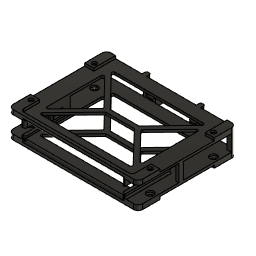
BatteryCase (Autodesk Fusion 360 design; units mm, degrees)
Autodesk Fusion 360 part; units mm, degrees
note: some values were not read from the file. Set by a fixed rule: the direction of a hole.
sketch "草图1" plane through (0, 0, 0) normal (0, 1, 0) x (1, 0, 0)
  line L0 (43, -8.75) -> (-43, -8.75)
  line L1 (-43, -8.75) -> (-43, 8.75)
  line L2 (-43, 8.75) -> (43, 8.75)
  line L3 (43, 8.75) -> (43, -8.75)
  line L4 (43, -8.75) -> (-43, 8.75) construction
  line L5 (-43, -8.75) -> (43, 8.75) construction
  dimension "d1" = 86
  dimension "d2" = 17.5
  constraint horizontal L0
  constraint perpendicular L0 L1
  constraint parallel L0 L2
  constraint parallel L1 L3
  constraint coincident L4 origin
  constraint coincident L5 origin
  measures "d1" distance of L1 L3
  measures "d2" distance of L0 L2
extrude "拉伸1" add sketch "草图1" along normal mid plane 65
sketch "草图2" plane through (0, -32.5, 0) normal (0, -1, 0) x (1, 0, 0)
  line L0 (-43, -8.75) -> (43, -8.75)
  line L1 (43, -8.75) -> (43, 8.75)
  line L2 (43, 8.75) -> (-43, 8.75)
  line L3 (-43, 8.75) -> (-43, -8.75)
  line L4 (32.075, 5.4) -> (-32.075, 5.4)
  line L5 (-32.075, 5.4) -> (-32.075, -5.4)
  line L6 (-32.075, -5.4) -> (32.075, -5.4)
  line L7 (32.075, -5.4) -> (32.075, 5.4)
  line L8 (32.075, 5.4) -> (-32.075, -5.4) construction
  line L9 (-32.075, 5.4) -> (32.075, -5.4) construction
  line L10 (0, 17) -> (0, -17) construction
  dimension "d5" = 64.15
  dimension "d6" = 10.8
  constraint horizontal L4
  constraint perpendicular L4 L5
  constraint parallel L4 L6
  constraint parallel L5 L7
  constraint perpendicular L0 L10
  constraint midpoint L8 origin
  constraint coincident L10 origin
  constraint coincident origin L10
  measures "d5" distance of L5 L7
  measures "d6" distance of L4 L6
extrude "拉伸2" cut sketch "草图2" against normal blind 85 contours L4 L5 L6 L7
sketch "草图3" plane through (-32.075, 0, 0) normal (1, 0, 0) x (0, 1, 0)
  line L0 (-32.5, 5.4) -> (-32.5, -5.4)
  line L1 (-32.5, -5.4) -> (32.5, -5.4)
  line L2 (32.5, -5.4) -> (32.5, 5.4)
  line L3 (32.5, 5.4) -> (-32.5, 5.4)
  line L4 (-32.5, 1.45) -> (-14.9, 1.45)
  line L5 (-14.9, 1.45) -> (-14.9, -2.95)
  line L6 (-14.9, -2.95) -> (-32.5, -2.95)
  line L7 (-32.5, -2.95) -> (-32.5, 1.45)
  line L8 (-7.4, 1.45) -> (-12.5, 1.45)
  line L9 (-12.5, 1.45) -> (-12.5, -2.95)
  line L10 (-12.5, -2.95) -> (-7.4, -2.95)
  line L11 (-7.4, -2.95) -> (-7.4, 1.45)
  dimension "d12" = 17.6
  dimension "d15" = 5.1
  dimension "d16" = 25.1
  dimension "d248" = 2.45
  dimension "d249" = 3.95
  constraint horizontal L4
  constraint vertical L5
  constraint horizontal L6
  constraint vertical L7
  constraint coincident L0 L4.start
  constraint horizontal L8
  constraint vertical L9
  constraint horizontal L10
  constraint vertical L11
  constraint collinear L4 L8
  constraint collinear L6 L10
  measures "d12" distance of L5 L7
  measures "d15" distance of L9 L11
  measures "d16" distance of L7 L11
  measures "d248" distance of L1 L10
  measures "d249" distance of L3 L4
extrude "拉伸3" cut sketch "草图3" along normal mid plane 170 contours L0 L4 L5 L6 L7 | L8 L9 L10 L11
sketch "草图15" plane through (0, -32.5, 0) normal (0, -1, 0) x (1, 0, 0)
  line L0 (32.075, 1.45) -> (43, 1.45)
  line L1 (43, 1.45) -> (43, 8.75)
  line L2 (43, 8.75) -> (-43, 8.75)
  line L3 (-43, 8.75) -> (-43, 1.45)
  line L4 (-43, 1.45) -> (-32.075, 1.45)
  line L5 (-32.075, 1.45) -> (-32.075, 5.4)
  line L6 (-32.075, 5.4) -> (32.075, 5.4)
  line L7 (32.075, 5.4) -> (32.075, 1.45)
  line L8 (-43, 5.8) -> (-34.075, 5.8)
  line L9 (-34.075, 5.8) -> (-34.075, -5.4)
  line L10 (-34.075, -5.4) -> (-43, -5.4)
  line L11 (-43, -5.4) -> (-43, 5.8)
  line L12 (-32.075, -5.4) -> (-32.075, -2.95)
  line L13 (32.075, -5.4) -> (-32.075, -5.4)
  line L14 (0, 15) -> (0, -16) construction
  line L15 (43, 5.8) -> (34.075, 5.8)
  line L16 (43, -5.4) -> (43, 5.8)
  line L17 (34.075, 5.8) -> (34.075, -5.4)
  line L18 (34.075, -5.4) -> (43, -5.4)
  line L19 (-43, -8.75) -> (43, -8.75)
  dimension "d153" = 2
  dimension "d162" = 2.95
  dimension "d163" = 3.35
  constraint horizontal L8
  constraint vertical L9
  constraint horizontal L10
  constraint vertical L11
  constraint coincident L3 L8.start
  constraint vertical L14
  constraint symmetric L8.start L14 L15.start
  constraint symmetric L8.end L14 L15.end
  constraint symmetric L9.end L14 L17.end
  constraint symmetric L10.end L14 L16.start
  measures "d153" distance of L9 L12
  measures "d162" distance of L2 L8
  measures "d163" distance of L10 L19
extrude "拉伸14" cut sketch "草图15" against normal blind 27 contours L0 L1 L15 L16 L17 | L0 L16 L17 L18 | L4 L9 L10 L11 | L3 L4 L8 L9 L11
sketch "草图16" plane through (-43, 0, 0) normal (-1, 0, 0) x (0, -1, 0)
  line L0 (5.5, 5.8) -> (32.5, 5.8)
  line L1 (32.5, 5.8) -> (32.5, 8.75)
  line L2 (32.5, 8.75) -> (-32.5, 8.75)
  line L3 (-32.5, 8.75) -> (-32.5, -8.75)
  line L4 (-32.5, -8.75) -> (32.5, -8.75)
  line L5 (32.5, -8.75) -> (32.5, -5.4)
  line L6 (32.5, -5.4) -> (5.5, -5.4)
  line L7 (5.5, -5.4) -> (5.5, 5.8)
  line L8 (-29.5, 5.4) -> (2.5, 5.4)
  line L9 (2.5, 5.4) -> (2.5, -5.4)
  line L10 (2.5, -5.4) -> (-29.5, -5.4)
  line L11 (-29.5, -5.4) -> (-29.5, 5.4)
  dimension "d156" = 3
  dimension "d157" = 3.35
  dimension "d158" = 3.35
  dimension "d159" = 3
  constraint horizontal L8
  constraint vertical L9
  constraint horizontal L10
  constraint vertical L11
  measures "d156" distance of L3 L11
  measures "d157" distance of L4 L10
  measures "d158" distance of L2 L8
  measures "d159" distance of L7 L9
extrude "拉伸15" cut sketch "草图16" against normal blind 86 contours L8 L9 L10 L11
sketch "草图4" plane through (0, 0, -5.4) normal (0, 0, -1) x (1, 0, 0)
  line L0 (-43, 30) -> (-43, -30)
  line L1 (-43, -30) -> (43, -30)
  line L2 (43, -30) -> (43, 30)
  line L3 (43, 30) -> (-43, 30)
  line L4 (-39.5, 21) -> (39.5, 21) construction
  line L5 (39.5, 21) -> (39.5, -21) construction
  line L6 (39.5, -21) -> (-39.5, -21) construction
  line L7 (-39.5, -21) -> (-39.5, 21) construction
  circle A0 centre (-39.5, 21) radius 2.35
  circle A1 centre (39.5, 21) radius 2.35
  circle A2 centre (-39.5, -21) radius 2.35
  circle A3 centre (39.5, -21) radius 2.35
  line L8 (35.05, -30) -> (-35.05, -30)
  line L9 (-35.05, -30) -> (-35.05, 30)
  line L10 (-35.05, 30) -> (35.05, 30)
  line L11 (35.05, 30) -> (35.05, -30)
  line L12 (-35.05, 30) -> (-35.05, 7.4)
  line L13 (-35.05, 7.4) -> (-36.55, 7.4)
  line L14 (-36.55, 30) -> (-35.05, 30)
  line L15 (-36.55, 7.4) -> (-36.55, 30)
  line L16 (-35.05, -4) -> (-35.05, -27)
  line L17 (-35.05, -27) -> (-43, -27)
  line L18 (-43, -27) -> (-43, -4)
  line L19 (-43, -4) -> (-35.05, -4)
  line L20 (-43, 32.5) -> (-34.075, 32.5)
  line L21 (-34.075, 32.5) -> (-34.075, 5.5)
  line L22 (-34.075, 5.5) -> (-43, 5.5)
  line L23 (-43, 5.5) -> (-43, 32.5)
  dimension "d17" = 79
  dimension "d18" = 42
  dimension "d19" = 39.5
  dimension "d20" = 21
  dimension "d21" = 4.7
  dimension "d22" = 4.7
  dimension "d23" = 4.7
  dimension "d24" = 4.7
  constraint horizontal L4
  constraint vertical L5
  constraint horizontal L6
  constraint vertical L7
  constraint coincident L4.start L7.end
  constraint coincident L4.end L5.start
  constraint coincident L6.end L7.start
  constraint coincident L5.end L6.start
  measures "d17" distance of L5 L7
  measures "d18" distance of L4 L6
  measures "d19" distance of origin L7
  measures "d20" distance of origin L4
  measures "d21" diameter of A0
  measures "d22" diameter of A1
  measures "d23" diameter of A2
  measures "d24" diameter of A3
extrude "拉伸20" cut sketch "草图4" along normal blind 1 contours A0 | A1 | A2 | A3
sketch "草图21" plane through (0, 0, -6.4) normal (0, 0, -1) x (1, 0, 0)
  circle A0 centre (-39.5, -21) radius 2.35
  point P0 (-39.5, -21)
  point P1 (-39.5, 21)
  point P2 (39.5, 21)
  point P3 (39.5, -21)
hole "孔2" at (-39.5, 21, -6.4) at (-39.5, -21, -6.4) at (39.5, -21, -6.4) at (39.5, 21, -6.4) direction (0, 0, -1) diameter 3.1 depth 3 tip angle 180 countersink diameter 4.7 countersink angle 90
sketch "草图10" plane through (0, 0, 5.8) normal (0, 0, -1) x (1, 0, 0)
  line L0 (-35.05, -30) -> (35.05, -30)
  line L1 (35.05, -30) -> (35.05, 30)
  line L2 (35.05, 30) -> (-35.05, 30)
  line L3 (-35.05, 30) -> (-35.05, -30)
  line L4 (-34.075, 32.5) -> (-43, 32.5)
  line L5 (-43, 32.5) -> (-43, 5.5)
  line L6 (-43, 5.5) -> (-34.075, 5.5)
  line L7 (-34.075, 5.5) -> (-34.075, 32.5)
  circle A0 centre (-39.5, 21) radius 2.35
  circle A1 centre (-39.5, -21) radius 2.35
  circle A2 centre (39.5, 21) radius 2.35
  circle A3 centre (39.5, -21) radius 2.35
  point P0 (-39.5, 21)
  point P1 (-39.5, -21)
  point P2 (39.5, -21)
  point P3 (39.5, 21)
  dimension "d206" = 4.7
  dimension "d207" = 4.7
  dimension "d208" = 4.7
  dimension "d209" = 4.7
  constraint coincident P0 A0.centre
  constraint coincident P1 A1.centre
  constraint coincident P3 A2.centre
  constraint coincident P2 A3.centre
  measures "d206" diameter of A0
  measures "d207" diameter of A2
  measures "d208" diameter of A3
  measures "d209" diameter of A1
extrude "拉伸21" cut sketch "草图10" against normal blind 1 contours A0 | A1 | A2 | A3
sketch "草图22" plane through (0, 0, 6.8) normal (0, 0, -1) x (1, 0, 0)
  circle A0 centre (39.5, -21) radius 2.35
  point P0 (-39.5, 21)
  point P1 (-39.5, -21)
  point P2 (39.5, 21)
  point P3 (39.5, -21)
  constraint coincident P3 A0.centre
hole "孔3" at (39.5, 21, 6.8) at (39.5, -21, 6.8) at (-39.5, -21, 6.8) at (-39.5, 21, 6.8) direction (0, 0, 1) diameter 3.1 depth 2 tip angle 180 countersink diameter 4.7 countersink angle 90
sketch "草图5" plane through (0, 0, -8.75) normal (0, 0, -1) x (1, 0, 0)
  line L0 (-43, 32.5) -> (-43, -32.5)
  line L1 (-43, -32.5) -> (43, -32.5)
  line L2 (43, -32.5) -> (43, 32.5)
  line L3 (43, 32.5) -> (-43, 32.5)
  line L4 (-29.472, -24.5) -> (29.2627, -24.5)
  line L5 (29.9836, -22.807) -> (9.5, -1.5)
  line L6 (9.5, -1.5) -> (-9.5, -1.5)
  line L7 (-9.5, -1.5) -> (-30.1894, -22.8033)
  line L8 (-47, 0) -> (46, 0) construction
  arc A0 (-30.1894, -22.8033) -> (-29.472, -24.5) centre (-29.472, -23.5) ccw
  arc A1 (29.2627, -24.5) -> (29.9836, -22.807) centre (29.2627, -23.5) ccw
  arc A2 (-29.472, 24.5) -> (-30.1894, 22.8033) centre (-29.472, 23.5) ccw
  line L9 (-29.472, 24.5) -> (29.2627, 24.5)
  arc A3 (29.9836, 22.807) -> (29.2627, 24.5) centre (29.2627, 23.5) ccw
  line L10 (29.9836, 22.807) -> (9.5, 1.5)
  line L11 (-9.5, 1.5) -> (-30.1894, 22.8033)
  line L12 (9.5, 1.5) -> (-9.5, 1.5)
  line L13 (-32.075, -17.9738) -> (-32.075, 17.9738)
  line L14 (-30.3576, 18.6705) -> (-12.9018, 0.6967)
  line L15 (-30.3576, -18.6705) -> (-12.9018, -0.6967)
  arc A4 (-32.075, -17.9738) -> (-30.3576, -18.6705) centre (-31.075, -17.9738) ccw
  arc A5 (-30.3576, 18.6705) -> (-32.075, 17.9738) centre (-31.075, 17.9738) ccw
  arc A6 (-12.9018, -0.6967) -> (-12.9018, 0.6967) centre (-13.6192, 0) ccw
  line L16 (0, -32) -> (0, 32) construction
  arc A7 (12.9018, 0.6967) -> (12.9018, -0.6967) centre (13.6192, 0) ccw
  line L17 (30.3576, -18.6705) -> (12.9018, -0.6967)
  arc A8 (30.3576, -18.6705) -> (32.075, -17.9738) centre (31.075, -17.9738) ccw
  line L18 (32.075, -17.9738) -> (32.075, 17.9738)
  line L19 (30.3576, 18.6705) -> (12.9018, 0.6967)
  arc A9 (32.075, 17.9738) -> (30.3576, 18.6705) centre (31.075, 17.9738) ccw
  circle A10 centre (39.5, 21) radius 1.55
  circle A11 centre (-39.5, -21) radius 1.55
  circle A12 centre (-39.5, 21) radius 1.55
  circle A13 centre (39.5, -21) radius 1.55
  point P0 (-31.8372, -24.5)
  point P1 (31.6112, -24.5)
  point P2 (0, -1.5)
  dimension "d164" = 8
  dimension "d165" = 1.5
  dimension "d168" = 19
  dimension "d169" = 1
  dimension "d170" = 3
  dimension "d171" = 10.925
  dimension "d172" = 1
  dimension "d173" = 1
  dimension "d174" = 1
  dimension "d175" = 3
  constraint horizontal L4
  constraint parallel L4 L6
  constraint coincident L6 P2
  constraint midpoint L6 P2
  constraint vertical origin P2
  constraint perpendicular L2 L8
  constraint coincident P0 L4
  constraint coincident P0 L7
  constraint tangent L4 A0
  constraint tangent L7 A0
  constraint coincident P1 L4
  constraint coincident P1 L5
  constraint tangent L4 A1
  constraint tangent L5 A1
  constraint equal A0 A1
  constraint symmetric L5.end L8 L10.end
  constraint symmetric L6.end L8 L11.start
  constraint symmetric L8 L4.start A2.start
  constraint symmetric L8 L7.end A2.end
  constraint symmetric L8 A0 A2
  constraint symmetric L8 L4.end L9.end
  constraint symmetric L8 L5.start A3.start
  constraint symmetric L8 A1 A3
  constraint perpendicular L8 L13
  constraint parallel L7 L15
  constraint parallel L11 L14
  constraint tangent L13 A4
  constraint tangent L15 A4
  constraint tangent L13 A5
  constraint tangent L14 A5
  constraint tangent L14 A6
  constraint tangent L15 A6
  constraint perpendicular L3 L16
  constraint symmetric L13.start L16 A8.end
  constraint symmetric L15.start L16 L17.start
  constraint symmetric A4 L16 A8
  constraint symmetric L13.end L16 L18.end
  constraint symmetric L14.start L16 L19.start
  constraint symmetric A5 L16 A9
  constraint symmetric L14.end L16 A7.start
  constraint symmetric L15.end L16 A7.end
  constraint symmetric A6 L16 A7
  measures "d164" distance of L1 L4
  measures "d165" distance of origin L6
  measures "d168" distance of L5.end L6.end
  measures "d169" radius of A0
  measures "d170" distance of L7 L15
  measures "d171" distance of L0 L13
  measures "d172" radius of A4
  measures "d173" radius of A5
  measures "d174" radius of A6
  measures "d175" distance of L11 L14
extrude "拉伸5" cut sketch "草图5" against normal blind 25 contours L4 L5 L6 L7 A0 A1 | A2 L9 A3 L10 L11 L12 | L13 L14 L15 A4 A5 A6 | A7 L17 A8 L18 L19 A9
sketch "草图6" plane through (0, 0, -8.75) normal (0, 0, -1) x (1, 0, 0)
  line L0 (-43, 32.5) -> (-43, -32.5)
  line L1 (-43, -32.5) -> (43, -32.5)
  line L2 (43, -32.5) -> (43, 32.5)
  line L3 (43, 32.5) -> (-43, 32.5)
  circle A0 centre (14, -36.5) radius 1.05
  circle A1 centre (-14, -36.5) radius 1.05
  line L4 (0, -40.5) -> (0, -15.5) construction
  line L5 (16.5, -40) -> (11.5, -40)
  line L6 (11.5, -40) -> (11.5, -32.5)
  line L7 (11.5, -32.5) -> (16.5, -32.5)
  line L8 (16.5, -32.5) -> (16.5, -40)
  line L9 (-16.5, -32.5) -> (-16.5, -40)
  line L10 (-16.5, -40) -> (-11.5, -40)
  line L11 (-11.5, -40) -> (-11.5, -32.5)
  line L12 (-11.5, -32.5) -> (-16.5, -32.5)
  line L13 (32.075, 17.9738) -> (32.075, -17.9738)
  arc A2 (30.3576, -18.6705) -> (32.075, -17.9738) centre (31.075, -17.9738) ccw
  line L14 (30.3576, -18.6705) -> (12.9018, -0.6967)
  arc A3 (12.9018, 0.6967) -> (12.9018, -0.6967) centre (13.6192, 0) ccw
  line L15 (12.9018, 0.6967) -> (30.3576, 18.6705)
  arc A4 (32.075, 17.9738) -> (30.3576, 18.6705) centre (31.075, 17.9738) ccw
  line L16 (-29.472, 24.5) -> (29.2627, 24.5)
  arc A5 (29.9836, 22.807) -> (29.2627, 24.5) centre (29.2627, 23.5) ccw
  line L17 (29.9836, 22.807) -> (9.5, 1.5)
  line L18 (9.5, 1.5) -> (-9.5, 1.5)
  line L19 (-9.5, 1.5) -> (-30.1894, 22.8033)
  arc A6 (-29.472, 24.5) -> (-30.1894, 22.8033) centre (-29.472, 23.5) ccw
  line L20 (9.5, -1.5) -> (29.9836, -22.807)
  arc A7 (29.2627, -24.5) -> (29.9836, -22.807) centre (29.2627, -23.5) ccw
  line L21 (29.2627, -24.5) -> (-29.472, -24.5)
  arc A8 (-30.1894, -22.8033) -> (-29.472, -24.5) centre (-29.472, -23.5) ccw
  line L22 (-30.1894, -22.8033) -> (-9.5, -1.5)
  line L23 (-9.5, -1.5) -> (9.5, -1.5)
  line L24 (-12.9018, -0.6967) -> (-30.3576, -18.6705)
  arc A9 (-32.075, -17.9738) -> (-30.3576, -18.6705) centre (-31.075, -17.9738) ccw
  line L25 (-32.075, -17.9738) -> (-32.075, 17.9738)
  arc A10 (-30.3576, 18.6705) -> (-32.075, 17.9738) centre (-31.075, 17.9738) ccw
  line L26 (-30.3576, 18.6705) -> (-12.9018, 0.6967)
  arc A11 (-12.9018, -0.6967) -> (-12.9018, 0.6967) centre (-13.6192, 0) ccw
  circle A12 centre (39.5, 21) radius 1.55
  circle A13 centre (-39.5, -21) radius 1.55
  circle A14 centre (-39.5, 21) radius 1.55
  circle A15 centre (39.5, -21) radius 1.55
  dimension "d33" = 2.1
  dimension "d34" = 2.1
  dimension "d35" = 14
  dimension "d36" = 14
  dimension "d37" = 4
  dimension "d38" = 3.5
  dimension "d39" = 2.5
  dimension "d40" = 2.5
  constraint horizontal A0.centre A1.centre
  constraint horizontal L5
  constraint vertical L6
  constraint horizontal L7
  constraint vertical L8
  constraint coincident L1 L6.end
  constraint symmetric L4 L5.start L9.end
  constraint symmetric L4 L5.end L10.end
  constraint symmetric L4 L6.end L11.end
  constraint symmetric L4 L7.end L9.start
  measures "d33" diameter of A0
  measures "d34" diameter of A1
  measures "d35" distance of A0.centre L4
  measures "d36" distance of A1.centre L4
  measures "d37" distance of L1 A0.centre
  measures "d38" distance of A0.centre L5
  measures "d39" distance of A0.centre L6
  measures "d40" distance of A0.centre L8
extrude "拉伸6" add sketch "草图6" against normal blind 5.3 contours L1 L9 L10 L11 L12 | L1 L5 L6 L7 L8
sketch "草图26" plane through (0, 0, -3.45) normal (0, 0, 1) x (-1, 0, 0)
  line L0 (-11.5, -32.5) -> (-16.5, -32.5)
  line L1 (-16.5, -32.5) -> (-16.5, -40)
  line L2 (-16.5, -40) -> (-11.5, -40)
  line L3 (-11.5, -40) -> (-11.5, -32.5)
  circle A0 centre (-14, -36.5) radius 2.05
  circle A1 centre (14, -36.5) radius 2.05
  point P0 (-14, -36.5)
  dimension "d229" = 28
  dimension "d230" = 4.1
  dimension "d231" = 4.1
  constraint coincident P0 A0.centre
  measures "d229" distance of P0 A1.centre
  measures "d230" diameter of A0
  measures "d231" diameter of A1
extrude "拉伸25" cut sketch "草图26" against normal blind 1.5 contours A0 | A1
sketch "草图12" plane through (0, 0, -8.75) normal (0, 0, -1) x (1, 0, 0)
  circle A0 centre (14, -36.5) radius 1.05
  line L0 (16.5, -40) -> (16.5, -32.5)
  line L1 (-11.5, -32.5) -> (11.5, -32.5)
  line L2 (43, -32.5) -> (43, 32.5)
  line L3 (-43, 32.5) -> (-43, -32.5)
  line L4 (-43, -32.5) -> (-16.5, -32.5)
  line L5 (-16.5, -32.5) -> (-16.5, -40)
  line L6 (-16.5, -40) -> (-11.5, -40)
  line L7 (-11.5, -40) -> (-11.5, -32.5)
  line L8 (11.5, -32.5) -> (11.5, -40)
  line L9 (11.5, -40) -> (16.5, -40)
  circle A1 centre (14, -36.5) radius 2
  circle A2 centre (-14, -36.5) radius 2
  line L10 (16.5, -32.5) -> (43, -32.5)
  line L11 (32.075, 17.9738) -> (32.075, -17.9738)
  arc A3 (30.3576, -18.6705) -> (32.075, -17.9738) centre (31.075, -17.9738) ccw
  line L12 (30.3576, -18.6705) -> (12.9018, -0.6967)
  arc A4 (12.9018, 0.6967) -> (12.9018, -0.6967) centre (13.6192, 0) ccw
  line L13 (12.9018, 0.6967) -> (30.3576, 18.6705)
  arc A5 (32.075, 17.9738) -> (30.3576, 18.6705) centre (31.075, 17.9738) ccw
  line L14 (-29.472, 24.5) -> (29.2627, 24.5)
  arc A6 (29.9836, 22.807) -> (29.2627, 24.5) centre (29.2627, 23.5) ccw
  line L15 (29.9836, 22.807) -> (9.5, 1.5)
  line L16 (9.5, 1.5) -> (-9.5, 1.5)
  line L17 (-9.5, 1.5) -> (-30.1894, 22.8033)
  arc A7 (-29.472, 24.5) -> (-30.1894, 22.8033) centre (-29.472, 23.5) ccw
  line L18 (9.5, -1.5) -> (29.9836, -22.807)
  arc A8 (29.2627, -24.5) -> (29.9836, -22.807) centre (29.2627, -23.5) ccw
  line L19 (29.2627, -24.5) -> (-29.472, -24.5)
  arc A9 (-30.1894, -22.8033) -> (-29.472, -24.5) centre (-29.472, -23.5) ccw
  line L20 (-30.1894, -22.8033) -> (-9.5, -1.5)
  line L21 (-9.5, -1.5) -> (9.5, -1.5)
  line L22 (-12.9018, -0.6967) -> (-30.3576, -18.6705)
  arc A10 (-32.075, -17.9738) -> (-30.3576, -18.6705) centre (-31.075, -17.9738) ccw
  line L23 (-32.075, -17.9738) -> (-32.075, 17.9738)
  arc A11 (-30.3576, 18.6705) -> (-32.075, 17.9738) centre (-31.075, 17.9738) ccw
  line L24 (-30.3576, 18.6705) -> (-12.9018, 0.6967)
  arc A12 (-12.9018, -0.6967) -> (-12.9018, 0.6967) centre (-13.6192, 0) ccw
  line L25 (43, 32.5) -> (-43, 32.5)
  circle A13 centre (-14, -36.5) radius 1.05
  circle A14 centre (39.5, 21) radius 1.55
  circle A15 centre (-39.5, -21) radius 1.55
  circle A16 centre (-39.5, 21) radius 1.55
  circle A17 centre (39.5, -21) radius 1.55
  dimension "d117" = 4
  dimension "d118" = 4
  constraint concentric A0 A1
  constraint concentric A2 A13
  measures "d117" diameter of A1
  measures "d118" diameter of A2
extrude "拉伸11" cut sketch "草图12" against normal blind 2 contours A1 | A2
sketch "草图27" plane through (0, 0, -6.75) normal (0, 0, -1) x (1, 0, 0)
  circle A0 centre (14, -36.5) radius 1.05
  circle A1 centre (14, -36.5) radius 2
  point P0 (14, -36.5)
  point P1 (-14, -36.5)
  constraint coincident P0 A0.centre
hole "孔4" at (14, 36.5, -6.75) at (-14, 36.5, -6.75) direction (0, 0, 1) diameter 2.1 depth 1.65 tip angle 118 countersink diameter 4 countersink angle 90
sketch "草图17" plane through (0, -2.5, 0) normal (0, 1, 0) x (-1, 0, 0)
  line L0 (32.075, -5.4) -> (43, -5.4)
  line L1 (43, -5.4) -> (43, 5.4)
  line L2 (43, 5.4) -> (32.075, 5.4)
  line L3 (34.075, -2.95) -> (32.075, -2.95)
  line L4 (32.075, -2.95) -> (32.075, -5.4)
  line L5 (32.075, -5.4) -> (34.075, -5.4)
  line L6 (34.075, -5.4) -> (34.075, -2.95)
  line L7 (34.075, -2.95) -> (34.075, -5.4)
  line L8 (-34.075, -2.95) -> (-32.075, -2.95)
  line L9 (0, 10) -> (0, -10) construction
  line L10 (34.075, -2.95) -> (32.075, -2.95)
  line L11 (-34.075, -2.95) -> (-32.075, -2.95)
  line L12 (-34.075, -5.4) -> (-34.075, -2.95)
  line L13 (-32.075, -2.95) -> (-32.075, -5.4)
  line L14 (32.075, -2.95) -> (-34.075, -5.4)
  line L15 (-32.075, -5.4) -> (-34.075, -5.4)
  line L16 (32.075, 5.4) -> (32.075, -5.4)
  line L17 (32.075, -2.95) -> (34.075, -2.95)
  point P0 (-32.075, -5.4)
  constraint horizontal L3
  constraint vertical L4
  constraint horizontal L5
  constraint vertical L6
  constraint coincident L0.start L4.end
  constraint collinear L6 L7
  constraint collinear L3 L8
  constraint vertical L9
  constraint symmetric L0.start L9 P0
  constraint symmetric L3.start L9 L8.start
  constraint symmetric L3.end L9 L8.end
  constraint symmetric L5.end L9 L12.start
  constraint symmetric L8.end L9 L3.end
  constraint symmetric L8.start L9 L3.start
extrude "拉伸16" add sketch "草图17" along normal blind 21 contours L0 L3 L4 L5 L6 L7 L10 L16 L17 | L13 L14 L15
sketch "草图18" plane through (0, 0, 8.75) normal (0, 0, 1) x (-1, 0, 0)
  line L0 (37, -32.5) -> (-37, -32.5)
  line L1 (-37, -32.5) -> (-37, 28.5)
  line L2 (-35, 30.5) -> (35, 30.5)
  line L3 (37, 28.5) -> (37, -32.5)
  line L4 (-43, 32.5) -> (43, 32.5)
  line L5 (-43, 32.5) -> (-43, -32.5)
  line L6 (43, 32.5) -> (43, -32.5)
  line L7 (43, -32.5) -> (-43, -32.5)
  arc A0 (37, 28.5) -> (35, 30.5) centre (35, 28.5) ccw
  arc A1 (-35, 30.5) -> (-37, 28.5) centre (-35, 28.5) ccw
  dimension "d217" = 2
  dimension "d218" = 6
  dimension "d219" = 6
  dimension "d220" = 2
  constraint horizontal L0
  constraint vertical L1
  constraint horizontal L2
  constraint vertical L3
  constraint collinear L0 L7
  constraint tangent L2 A0
  constraint tangent L3 A0
  constraint tangent L1 A1
  constraint tangent L2 A1
  constraint equal A0 A1
  measures "d217" distance of L2 L4
  measures "d218" distance of L1 L5
  measures "d219" distance of L3 L6
  measures "d220" radius of A0
extrude "拉伸17" cut sketch "草图18" against normal blind 1.75 contours L0 L1 L2 L3 L7 A0 A1
sketch "草图19" plane through (0, 0, -8.75) normal (0, 0, -1) x (1, 0, 0)
  circle A0 centre (14, -36.5) radius 2
  line L0 (32.075, 17.9738) -> (32.075, -17.9738)
  arc A1 (30.3576, -18.6705) -> (32.075, -17.9738) centre (31.075, -17.9738) ccw
  line L1 (30.3576, -18.6705) -> (12.9018, -0.6967)
  arc A2 (12.9018, 0.6967) -> (12.9018, -0.6967) centre (13.6192, 0) ccw
  line L2 (12.9018, 0.6967) -> (30.3576, 18.6705)
  arc A3 (32.075, 17.9738) -> (30.3576, 18.6705) centre (31.075, 17.9738) ccw
  line L3 (-29.472, 24.5) -> (29.2627, 24.5)
  arc A4 (29.9836, 22.807) -> (29.2627, 24.5) centre (29.2627, 23.5) ccw
  line L4 (29.9836, 22.807) -> (9.5, 1.5)
  line L5 (9.5, 1.5) -> (-9.5, 1.5)
  line L6 (-9.5, 1.5) -> (-30.1894, 22.8033)
  arc A5 (-29.472, 24.5) -> (-30.1894, 22.8033) centre (-29.472, 23.5) ccw
  line L7 (9.5, -1.5) -> (29.9836, -22.807)
  arc A6 (29.2627, -24.5) -> (29.9836, -22.807) centre (29.2627, -23.5) ccw
  line L8 (29.2627, -24.5) -> (-29.472, -24.5)
  arc A7 (-30.1894, -22.8033) -> (-29.472, -24.5) centre (-29.472, -23.5) ccw
  line L9 (-30.1894, -22.8033) -> (-9.5, -1.5)
  line L10 (-9.5, -1.5) -> (9.5, -1.5)
  line L11 (-12.9018, -0.6967) -> (-30.3576, -18.6705)
  arc A8 (-32.075, -17.9738) -> (-30.3576, -18.6705) centre (-31.075, -17.9738) ccw
  line L12 (-32.075, -17.9738) -> (-32.075, 17.9738)
  arc A9 (-30.3576, 18.6705) -> (-32.075, 17.9738) centre (-31.075, 17.9738) ccw
  line L13 (-30.3576, 18.6705) -> (-12.9018, 0.6967)
  arc A10 (-12.9018, -0.6967) -> (-12.9018, 0.6967) centre (-13.6192, 0) ccw
  line L14 (-43, 32.5) -> (-43, -32.5)
  line L15 (-43, -32.5) -> (-16.5, -32.5)
  line L16 (-16.5, -32.5) -> (-16.5, -40)
  line L17 (-16.5, -40) -> (-11.5, -40)
  line L18 (-11.5, -40) -> (-11.5, -32.5)
  line L19 (-11.5, -32.5) -> (11.5, -32.5)
  line L20 (11.5, -32.5) -> (11.5, -40)
  line L21 (11.5, -40) -> (16.5, -40)
  line L22 (16.5, -40) -> (16.5, -32.5)
  line L23 (16.5, -32.5) -> (43, -32.5)
  line L24 (43, -32.5) -> (43, 32.5)
  line L25 (43, 32.5) -> (-43, 32.5)
  line L26 (-35, 29.5) -> (35, 29.5)
  line L27 (37, 27.5) -> (37, -27.5)
  line L28 (35, -29.5) -> (-35, -29.5)
  line L29 (-37, -27.5) -> (-37, 27.5)
  arc A11 (-35, 29.5) -> (-37, 27.5) centre (-35, 27.5) ccw
  arc A12 (-37, -27.5) -> (-35, -29.5) centre (-35, -27.5) ccw
  arc A13 (35, -29.5) -> (37, -27.5) centre (35, -27.5) ccw
  arc A14 (37, 27.5) -> (35, 29.5) centre (35, 27.5) ccw
  circle A15 centre (-14, -36.5) radius 2
  circle A16 centre (39.5, 21) radius 1.55
  circle A17 centre (-39.5, -21) radius 1.55
  circle A18 centre (-39.5, 21) radius 1.55
  circle A19 centre (39.5, -21) radius 1.55
  dimension "d190" = 6
  dimension "d191" = 6
  dimension "d192" = 3
  dimension "d193" = 3
  dimension "d194" = 2
  constraint horizontal L26
  constraint vertical L27
  constraint horizontal L28
  constraint vertical L29
  constraint tangent L26 A11
  constraint tangent L29 A11
  constraint tangent L28 A12
  constraint tangent L29 A12
  constraint equal A11 A12
  constraint tangent L27 A13
  constraint tangent L28 A13
  constraint equal A11 A13
  constraint tangent L26 A14
  constraint tangent L27 A14
  constraint equal A11 A14
  measures "d190" distance of L14 L29
  measures "d191" distance of L24 L27
  measures "d192" distance of L25 L26
  measures "d193" distance of L19 L28
  measures "d194" radius of A11
extrude "拉伸18" cut sketch "草图19" against normal blind 1.75 contours L26 L27 L28 L29 A11 A12 A13 A14
sketch "草图20" plane through (-43, 0, 0) normal (-1, 0, 0) x (0, -1, 0)
  line L0 (2.5, 5.4) -> (2.5, -5.4)
  line L1 (2.5, -5.4) -> (-29.5, -5.4)
  line L2 (-29.5, -5.4) -> (-29.5, 5.4)
  line L3 (-29.5, 5.4) -> (2.5, 5.4)
  line L4 (5.5, 5.8) -> (32.5, 5.8)
  line L5 (32.5, 5.8) -> (32.5, 8.75)
  line L6 (32.5, 8.75) -> (-32.5, 8.75)
  line L7 (-32.5, 8.75) -> (-32.5, -8.75)
  line L8 (-32.5, -8.75) -> (32.5, -8.75)
  line L9 (32.5, -8.75) -> (32.5, -5.4)
  line L10 (32.5, -5.4) -> (5.5, -5.4)
  line L11 (5.5, -5.4) -> (5.5, 5.8)
  line L12 (-18, -7) -> (18, -7)
  line L13 (18, -7) -> (18, -8.75)
  line L14 (18, -8.75) -> (-18, -8.75)
  line L15 (-18, -8.75) -> (-18, -7)
  line L16 (0, 0) -> (0, -13) construction
  line L17 (-29.5, -5.4) -> (-32.5, -5.4)
  line L18 (32.5, -5.4) -> (17.9738, -5.4)
  line L19 (-17.9738, -5.4) -> (-18.5, -5.4)
  dimension "d198" = 36
  dimension "d201" = 1.75
  constraint horizontal L12
  constraint vertical L13
  constraint horizontal L14
  constraint vertical L15
  constraint coincident L8 L13.end
  constraint coincident L16.start origin
  constraint parallel L11 L16
  constraint symmetric L13 L15 L16
  measures "d198" distance of L13 L15
  measures "d201" distance of L12 L14
extrude "拉伸19" cut sketch "草图20" against normal blind 86 contours L8 L12 L13 L14 L15
sketch "草图23" plane through (0, -5.5, 0) normal (0, -1, 0) x (1, 0, 0)
  line L0 (-43, -5.4) -> (-34.075, -5.4)
  line L1 (-34.075, 5.8) -> (-43, 5.8)
  line L2 (-43, 5.8) -> (-43, -5.4)
  line L3 (-41, 5.8) -> (-34.075, 5.8)
  line L4 (-34.075, 5.8) -> (-34.075, -5.4)
  line L5 (-34.075, -5.4) -> (-41, -5.4)
  line L6 (-41, -5.4) -> (-41, 5.8)
  line L7 (0, 15) -> (0, -11) construction
  line L8 (41, 5.8) -> (34.075, 5.8)
  line L9 (41, -5.4) -> (41, 5.8)
  line L10 (34.075, 5.8) -> (34.075, -5.4)
  line L11 (34.075, -5.4) -> (41, -5.4)
  line L12 (-34.075, -5.4) -> (-34.075, 5.8)
  dimension "d214" = 2
  constraint horizontal L3
  constraint vertical L4
  constraint horizontal L5
  constraint vertical L6
  constraint coincident L0.end L4.end
  constraint coincident L1 L3.start
  constraint vertical L7
  constraint symmetric L3.start L7 L8.start
  constraint symmetric L1.start L7 L8.end
  constraint symmetric L0.end L7 L10.end
  constraint symmetric L5.end L7 L9.start
  measures "d214" distance of L2 L6
extrude "拉伸22" cut sketch "草图23" against normal blind 3 contours L0 L1 L3 L4 L5 L6 L12 | L8 L9 L10 L11
sketch "草图24" plane through (0, 32.5, 0) normal (0, 1, 0) x (-1, 0, 0)
  line L0 (37, 8.75) -> (37, 7)
  line L1 (37, 7) -> (-37, 7)
  line L2 (-37, 7) -> (-37, 8.75)
  line L3 (-37, 8.75) -> (-43, 8.75)
  line L4 (-43, 8.75) -> (-43, -8.75)
  line L5 (-43, -8.75) -> (-16.5, -8.75)
  line L6 (-16.5, -8.75) -> (-16.5, -5.4)
  line L7 (-16.5, -5.4) -> (-32.075, -5.4)
  line L8 (-32.075, -5.4) -> (-32.075, 5.4)
  line L9 (-32.075, 5.4) -> (32.075, 5.4)
  line L10 (32.075, 5.4) -> (32.075, -5.4)
  line L11 (16.5, -5.4) -> (16.5, -8.75)
  line L12 (16.5, -8.75) -> (43, -8.75)
  line L13 (43, -8.75) -> (43, 8.75)
  line L14 (43, 8.75) -> (37, 8.75)
  line L15 (-40, 5.4) -> (40, 5.4)
  line L16 (40, 5.4) -> (40, -5.4)
  line L17 (40, -5.4) -> (-40, -5.4)
  line L18 (-40, -5.4) -> (-40, 5.4)
  line L19 (32.075, -5.4) -> (16.5, -5.4)
  dimension "d221" = 3
  dimension "d222" = 3
  constraint horizontal L15
  constraint vertical L16
  constraint horizontal L17
  constraint vertical L18
  constraint collinear L9 L15
  measures "d221" distance of L13 L16
  measures "d222" distance of L4 L18
extrude "拉伸23" cut sketch "草图24" against normal blind 35 contours L10 L15 L16 L17 | L8 L15 L17 L18
sketch "草图25" plane through (-43, 0, 0) normal (-1, 0, 0) x (0, -1, 0)
  line L0 (-18, -8.75) -> (-18, -7)
  line L1 (-18, -7) -> (18, -7)
  line L2 (18, -7) -> (18, -8.75)
  line L3 (18, -8.75) -> (32.5, -8.75)
  line L4 (32.5, -8.75) -> (32.5, -5.4)
  line L5 (32.5, -5.4) -> (5.5, -5.4)
  line L6 (5.5, -5.4) -> (5.5, 5.8)
  line L7 (5.5, 5.8) -> (32.5, 5.8)
  line L8 (32.5, 5.8) -> (32.5, 8.75)
  line L9 (32.5, 8.75) -> (-32.5, 8.75)
  line L10 (-32.5, 8.75) -> (-32.5, -8.75)
  line L11 (-32.5, -8.75) -> (-18, -8.75)
  line L12 (2.5, 5.4) -> (2.5, -5.4)
  line L13 (2.5, -5.4) -> (-29.5, -5.4)
  line L14 (-29.5, -5.4) -> (-29.5, 5.4)
  line L15 (-29.5, 5.4) -> (2.5, 5.4)
  line L16 (-18, 8.75) -> (18, 8.75)
  line L17 (18, 8.75) -> (18, 7)
  line L18 (18, 7) -> (-18, 7)
  line L19 (-18, 7) -> (-18, 8.75)
  line L20 (0, 12) -> (0, -10) construction
  dimension "d225" = 1.75
  dimension "d226" = 36
  constraint horizontal L16
  constraint vertical L17
  constraint horizontal L18
  constraint vertical L19
  constraint coincident L9 L16.start
  constraint perpendicular L1 L20
  constraint symmetric L17 L19 L20
  measures "d225" distance of L16 L18
  measures "d226" distance of L17 L19
extrude "拉伸24" cut sketch "草图25" against normal blind 86 contours L9 L16 L17 L18 L19
sketch "草图13" plane through (0, 0, -8.75) normal (0, 0, -1) x (1, 0, 0)
  line L0 (-43, -18) -> (-43, -32.5)
  line L1 (43, -32.5) -> (43, -18)
  line L2 (16.5, -32.5) -> (19.5, -32.5)
  line L3 (19.5, -32.5) -> (19.5, -35.5)
  line L4 (19.5, -35.5) -> (16.5, -35.5)
  line L5 (16.5, -35.5) -> (16.5, -32.5)
  line L6 (0, -40) -> (0, -20) construction
  line L7 (-19.5, -32.5) -> (-19.5, -35.5)
  line L8 (-19.5, -35.5) -> (-16.5, -35.5)
  line L9 (-16.5, -32.5) -> (-19.5, -32.5)
  line L10 (-16.5, -35.5) -> (-16.5, -32.5)
  circle A0 centre (14, -36.5) radius 2
  circle A1 centre (-14, -36.5) radius 2
  line L11 (-43, -32.5) -> (-16.5, -32.5)
  line L12 (-16.5, -32.5) -> (-16.5, -40)
  line L13 (-16.5, -40) -> (-11.5, -40)
  line L14 (-11.5, -40) -> (-11.5, -32.5)
  line L15 (-11.5, -32.5) -> (11.5, -32.5)
  line L16 (11.5, -32.5) -> (11.5, -40)
  line L17 (11.5, -40) -> (16.5, -40)
  line L18 (16.5, -40) -> (16.5, -32.5)
  line L19 (16.5, -32.5) -> (43, -32.5)
  line L20 (43, -18) -> (37, -18)
  line L21 (37, -18) -> (37, -27.5)
  arc A2 (35, -29.5) -> (37, -27.5) centre (35, -27.5) ccw
  line L22 (35, -29.5) -> (-35, -29.5)
  arc A3 (-37, -27.5) -> (-35, -29.5) centre (-35, -27.5) ccw
  line L23 (-37, -27.5) -> (-37, -18)
  line L24 (-37, -18) -> (-43, -18)
  circle A4 centre (-39.5, -21) radius 1.55
  circle A5 centre (39.5, -21) radius 1.55
  point P0 (-20, -30)
  dimension "d135" = 3
  dimension "d136" = 3
  constraint horizontal L2
  constraint vertical L3
  constraint horizontal L4
  constraint vertical L5
  constraint symmetric L2.start L6 L9.start
  constraint symmetric L2.end L6 L7.start
  constraint symmetric L3.end L6 L7.end
  constraint symmetric L4.end L6 L8.end
  constraint collinear L2 L19
  constraint collinear L5 L18
  measures "d135" distance of L2 L4
  measures "d136" distance of L3 L5
extrude "拉伸12" add sketch "草图13" against normal up to surface (15.75 mm away) contours L7 L8 L9 L10 L11 L12 | L2 L3 L4 L5 L18 L19
fillet "圆角3" radius 2 4 edges at (-16.5, 40, -6.1) (-11.5, 40, -6.1) (11.5, 40, -6.1) (16.5, 40, -6.1)
fillet "圆角5" radius 1 10 edges at (-19.5, 32.5, 0) (-19.5, 32.5, -7.075) (-19.5, 35.5, -0.875) (-16.5, 35.5, 1.775) (-16.5, 35.5, -6.1) (16.5, 35.5, 1.775) (16.5, 35.5, -6.1) (19.5, 35.5, -0.875) (19.5, 32.5, 0) (19.5, 32.5, -7.075)
fillet "圆角6" radius 3 6 edges at (-43, 32.5, 0) (43, 32.5, 0) (43, -32.5, -7.075) (43, -32.5, 7.275) (-43, -32.5, 7.275) (-43, -32.5, -7.075)
fillet "圆角8" radius 1 4 edges at (14, 32.5, -3.45) (11.5, 32.5, -4.425) (-11.5, 32.5, -4.425) (-14, 32.5, -3.45)
fillet "圆角8" radius 1 2 edges at (11.5, 32.5, -7.075) (-11.5, 32.5, -7.075)
fillet "圆角9" radius 1.5 6 edges at (0, -32.5, -5.4) (0, -32.5, 5.4) (-32.075, -32.5, -4.175) (-32.075, -32.5, 3.425) (32.075, -32.5, 3.425) (32.075, -32.5, -4.175)
chamfer "倒角1" distance 1 distance2 1 2 edges at (-32.075, -14.9, -0.75) (32.075, -14.9, -0.75) measured on face at (-32.075, -4.1333, 0.4833) measured on face at (32.075, -4.1333, 0.4833)
chamfer "倒角1" distance 1 distance2 1 2 edges at (-32.075, -12.5, -0.75) (32.075, -12.5, -0.75) measured on face at (-32.075, -4.1333, 0.4833) measured on face at (32.075, -4.1333, 0.4833)
sketch "草图28" plane through (0, -2.5, 0) normal (0, 1, 0) x (-1, 0, 0)
  line L0 (34.075, -5.4) -> (34.075, -2.95)
  line L1 (34.075, -2.95) -> (32.075, -2.95)
  line L2 (32.075, -2.95) -> (32.075, -5.4)
  line L3 (32.075, -5.4) -> (33.275, -5.4)
  line L4 (33.275, -5.4) -> (33.275, -4.2)
  line L5 (33.275, -4.2) -> (32.075, -4.2)
  line L6 (32.075, -4.2) -> (32.075, -5.4)
  line L7 (0, 0) -> (0, -11.6167) construction
  line L8 (-32.075, -5.4) -> (-33.275, -5.4)
  line L9 (-33.275, -4.2) -> (-32.075, -4.2)
  line L10 (-33.275, -5.4) -> (-33.275, -4.2)
  line L11 (-32.075, -4.2) -> (-32.075, -5.4)
  line L12 (32.075, -5.4) -> (34.075, -5.4)
  line L13 (34.075, -5.4) -> (34.075, 5.4)
  line L14 (34.075, 5.4) -> (32.075, 5.4)
  line L15 (32.075, 5.4) -> (32.075, -5.4)
  line L16 (32.075, -5.4) -> (34.075, -5.4)
  point P0 (-32.075, -5.4)
  dimension "d250" = 1.2
  dimension "d251" = 1.2
  constraint horizontal L3
  constraint vertical L4
  constraint horizontal L5
  constraint vertical L6
  constraint coincident L2.end L3.start
  constraint coincident L7.start origin
  constraint vertical L7
  constraint symmetric L2.end L7 P0
  constraint symmetric L3.end L7 L8.end
  constraint symmetric L4.end L7 L9.start
  constraint symmetric L5.end L7 L9.end
  measures "d250" distance of L4.end L5.end
  measures "d251" distance of L3.end L4.end
extrude "拉伸26" cut sketch "草图28" against normal blind 51 contours L2 L3 L4 L5 L6 L12 L15 L16 | L8 L9 L10 L11
fillet "圆角10" radius 1 2 edges at (-34.075, -17.5, -5.4) (34.075, -17.5, -5.4)
equation "d171 = 11 mm - 0.075 mm"
